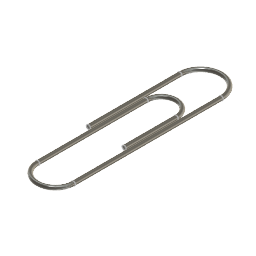
Day 3 - Paper Clip (Autodesk Fusion 360 design; units mm, degrees)
part number: 2025-06-14-22-08-39-769
Autodesk Fusion 360 part; units mm, degrees
sketch "Sweep Path" plane through (0, 0, 0) normal (0, 0, 1) x (1, 0, 0)
  line L0 (-0.0796, 0) -> (-0.0796, 16.25)
  line L1 (-0.0796, 16.25) -> (7.4204, 16.25) construction
  line L2 (7.4204, 16.25) -> (7.4204, -10)
  line L3 (7.4204, -10) -> (0.9204, -10) construction
  line L4 (0.9204, -10) -> (0.9204, 9.25)
  line L5 (0.9204, 9.25) -> (6.4204, 9.25) construction
  line L6 (6.4204, 9.25) -> (6.4204, 0)
  arc A0 (7.4204, 16.25) -> (-0.0796, 16.25) centre (3.6704, 16.25) ccw
  arc A1 (6.4204, 9.25) -> (0.9204, 9.25) centre (3.6704, 9.25) ccw
  arc A2 (0.9204, -10) -> (7.4204, -10) centre (4.1704, -10) ccw
  dimension "d14" = 16.25
  dimension "d15" = 7.5
  dimension "d16" = 26.25
  dimension "d17" = 6.5
  dimension "d18" = 19.25
  dimension "d19" = 5.5
  dimension "d20" = 9.25
  constraint vertical L0
  constraint perpendicular L0 L1
  constraint perpendicular L1 L2
  constraint perpendicular L2 L3
  constraint perpendicular L3 L4
  constraint perpendicular L2 L5
  constraint perpendicular L5 L6
  constraint tangent L0 A0
  constraint tangent L4 A1
  constraint tangent L4 A2
  measures "d14" distance of L0.start L0.end
  measures "d15" distance of L0.end L1.end
  measures "d16" distance of L1.end L2.end
  measures "d17" distance of L2.end L3.end
  measures "d18" distance of L3.end L4.end
  measures "d19" distance of L4.end L5.end
  measures "d20" distance of L5.end L6.end
sketch "Sweep Profile" plane through (0, 0, 0) normal (0, 1, 0) x (1, 0, 0)
  circle A0 centre (0, 0) radius 0.375
  dimension "d21" = 0.75
  constraint coincident A0.centre origin
  measures "d21" diameter of A0
sweep "Sweep1" add profiles "Sweep Profile" path "Sweep Path" along L0 A0 L2 A2 L4 A1 L6 section 1
